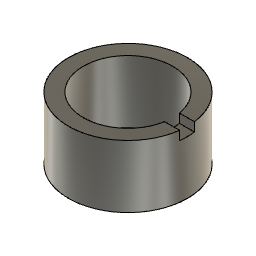
DC Motor Chuck Spacer v3 (Autodesk Fusion 360 design; units mm, degrees)
Autodesk Fusion 360 part; units mm, degrees
sketch "Sketch1" plane through (0, 0, 0) normal (0, 0, 1) x (1, 0, 0)
  circle A0 centre (0, 0) radius 15
  circle A1 centre (0, 0) radius 20
  dimension "d1" = 30
  dimension "d2" = 5
  constraint coincident A0.centre A1.centre
  measures "d1" diameter of A0
extrude "Extrude1" add sketch "Sketch1" along normal blind 21
sketch "Sketch2" plane through (0, 0, 21) normal (0, 0, 1) x (-1, 0, 0)
  circle A0 centre (0, 0) radius 15
  circle A1 centre (0, 0) radius 20
  line L0 (-14.7902, -2.5) -> (-19.8431, -2.5)
  line L1 (-14.7902, 2.5) -> (-19.8431, 2.5)
  line L2 (-14.7902, -2.5) -> (-14.7902, 2.5) construction
  point P0 (-14.7902, 0)
  dimension "d5" = 5
  constraint coincident A0 L0.start
  constraint coincident A1 L0.end
  constraint horizontal L0
  constraint coincident A0 L1.start
  constraint coincident A1 L1.end
  constraint parallel L0 L1
  constraint perpendicular L1 L2
  constraint midpoint L2 P0
  measures "d5" distance of L0 L1
extrude "Extrude2" cut sketch "Sketch2" against normal blind 3 contours A0 A1 L0 L1 picked at (-16.5367, -1.9456)
named bodies: "DC Motor Chuck Spacer"
